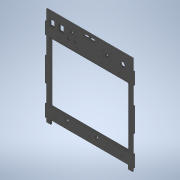
# Autodesk Inventor part: Frente Carcasa
Saved by Autodesk Inventor 2020 (Build 240168000, 168)
## iProperties
Created: 2020-06-04
Part Number: Frente Carcasa
Material: MDF Medium Density Fiberboard
Document SubType Name: Modeling
Designer: Dante
Density: 0.8 g/cm^3
Appearance: Gris oscuro
Mass: 813.806 g
Surface Area: 2644.18 cm^2
Volume: 1017.26 cm^3
Author: Dante
Autodesk Inventor part; units mm, degrees
ref_plane "YZ Plane" through (0, 0, 0) normal (1, 0, 0) x (0, 1, 0)
ref_plane "XZ Plane" through (0, 0, 0) normal (0, 1, 0) x (-1, 0, 0)
ref_plane "XY Plane" through (0, 0, 0) normal (0, 0, 1) x (1, 0, 0)
sketch "Sketch1" plane through (0, 0, 0) normal (0, 0, 1) x (1, 0, 0)
  line L0 (67.9652, 2.3975) -> (457.9652, 2.3975)
  line L1 (479.9652, -17.6025) -> (457.9652, -17.6025)
  line L2 (457.9652, -17.6025) -> (457.9652, 2.3975)
  line L3 (45.9652, -17.6025) -> (67.9652, -17.6025)
  line L4 (67.9652, -17.6025) -> (67.9652, 2.3975)
  line L5 (479.9652, 59.8925) -> (479.9652, 59.8925)
  line L6 (456.9652, 57.3975) -> (68.9652, 57.3975)
  line L7 (36.9652, 522.3965) -> (36.9552, 522.3965)
  line L8 (463.9652, 64.3975) -> (463.9652, 356.3975)
  line L9 (61.9652, 64.3975) -> (61.9652, 356.3975)
  line L10 (68.9652, 363.3975) -> (456.9652, 363.3975)
  line L11 (479.9652, 150.3975) -> (485.4652, 150.3975)
  line L12 (479.9652, 270.3975) -> (485.4652, 270.3975)
  line L13 (485.4652, 270.3975) -> (485.4652, 150.3975)
  line L14 (40.4652, 270.3975) -> (40.4652, 150.3975)
  line L15 (40.4652, 150.3975) -> (45.9652, 150.3975)
  line L16 (40.4652, 270.3975) -> (45.9652, 270.3975)
  circle A0 centre (95.9652, 27.3975) radius 3
  circle A1 centre (429.9652, 27.3975) radius 3
  circle A2 centre (417.4652, 381.0395) radius 3
  circle A3 centre (108.4652, 381.0395) radius 3
  circle A4 centre (327.4652, 381.0395) radius 3
  circle A5 centre (198.4652, 381.0395) radius 3
  circle A6 centre (262.9652, 27.3975) radius 3
  circle A7 centre (471.4652, 135.3975) radius 2
  circle A8 centre (471.4652, 285.3975) radius 2
  line L17 (45.9652, 270.3975) -> (45.9652, 360.3975)
  line L18 (45.9652, 360.3975) -> (40.4652, 360.3975)
  line L19 (40.4652, 360.3975) -> (40.4652, 420.3975)
  line L20 (40.4652, 420.3975) -> (45.9652, 420.3975)
  line L21 (45.9652, 475.4975) -> (45.9652, 420.3975)
  line L22 (45.9652, 360.3975) -> (45.9652, 270.3975)
  line L23 (45.9652, 150.3975) -> (45.9652, 60.3975)
  line L24 (45.9652, 60.3975) -> (40.4652, 60.3975)
  line L25 (40.4652, 60.3975) -> (40.4652, 0.3975)
  line L26 (40.4652, 0.3975) -> (45.9652, 0.3975)
  line L27 (45.9652, 150.3975) -> (45.9652, 60.3975)
  line L28 (45.9652, 0.3975) -> (45.9652, -17.6025)
  line L29 (479.9652, 360.3975) -> (485.4652, 360.3975)
  line L30 (485.4652, 360.3975) -> (485.4652, 420.3975)
  line L31 (485.4652, 420.3975) -> (479.9652, 420.3975)
  line L32 (479.9652, 475.4975) -> (479.9652, 420.3975)
  line L33 (479.9652, 150.3975) -> (479.9652, 60.3975)
  line L34 (479.9652, 60.3975) -> (485.4652, 60.3975)
  line L35 (485.4652, 60.3975) -> (485.4652, 0.3975)
  line L36 (485.4652, 0.3975) -> (479.9652, 0.3975)
  line L37 (479.9652, -17.6025) -> (479.9652, 0.3975)
  line L38 (479.9652, 60.3975) -> (479.9652, 150.3975)
  line L39 (479.9652, 270.3975) -> (479.9652, 360.3975)
  line L40 (262.9652, 474.8975) -> (262.9652, 460.6682)
  circle A9 centre (218.9652, 465.4975) radius 1.5
  circle A10 centre (218.9652, 400.4975) radius 1.5
  circle A11 centre (306.9652, 465.4975) radius 1.5
  circle A12 centre (306.9652, 400.4975) radius 1.5
  line L41 (266.4652, 463.3975) -> (290.7652, 463.3975)
  line L42 (290.7652, 463.3975) -> (290.7652, 450.7975)
  line L43 (290.7652, 450.7975) -> (266.4652, 450.7975)
  line L44 (266.4652, 450.7975) -> (266.4652, 463.3975)
  line L45 (235.4652, 463.3975) -> (259.7652, 463.3975)
  line L46 (259.7652, 463.3975) -> (259.7652, 450.7975)
  line L47 (259.7652, 450.7975) -> (235.4652, 450.7975)
  line L48 (235.4652, 450.7975) -> (235.4652, 463.3975)
  line L49 (86.9652, 440.4975) -> (65.4652, 440.4975)
  line L50 (65.4652, 440.4975) -> (65.4652, 414.9975)
  line L51 (65.4652, 414.9975) -> (86.9652, 414.9975)
  line L52 (86.9652, 414.9975) -> (86.9652, 440.4975)
  line L53 (87.0652, 441.9975) -> (87.0652, 413.4975)
  line L54 (65.3652, 413.4975) -> (65.3652, 441.9975)
  line L55 (133.4652, 440.4975) -> (111.9652, 440.4975)
  line L56 (111.9652, 440.4975) -> (111.9652, 414.9975)
  line L57 (111.9652, 414.9975) -> (133.4652, 414.9975)
  line L58 (133.4652, 414.9975) -> (133.4652, 440.4975)
  line L59 (133.5652, 441.9975) -> (133.5652, 413.4975)
  line L60 (111.8652, 413.4975) -> (111.8652, 441.9975)
  circle A13 centre (160.4652, 403.4975) radius 6
  circle A14 centre (175.4652, 435.4975) radius 6.5
  circle A15 centre (350.4652, 425.4975) radius 6.5
  circle A16 centre (193.4652, 448.4975) radius 2
  circle A17 centre (193.4652, 422.4975) radius 2
  circle A18 centre (157.4652, 448.4975) radius 2
  circle A19 centre (157.4652, 422.4975) radius 2
  circle A20 centre (368.4652, 438.4975) radius 2
  circle A21 centre (368.4652, 412.4975) radius 2
  circle A22 centre (332.4652, 438.4975) radius 2
  circle A23 centre (332.4652, 412.4975) radius 2
  circle A24 centre (429.9652, 425.4975) radius 11
  circle A25 centre (190.4652, 403.4975) radius 4.125
  line L61 (45.9652, 475.4975) -> (479.9652, 475.4975)
  line L62 (65.3652, 441.9975) -> (87.0652, 441.9975)
  line L63 (65.3652, 413.4975) -> (87.0652, 413.4975)
  line L64 (111.8652, 441.9975) -> (133.5652, 441.9975)
  line L65 (111.8652, 413.4975) -> (133.5652, 413.4975)
  arc A26 (68.9652, 363.3975) -> (61.9652, 356.3975) centre (68.9652, 356.3975) ccw
  arc A27 (61.9652, 64.3975) -> (68.9652, 57.3975) centre (68.9652, 64.3975) ccw
  arc A28 (456.9652, 57.3975) -> (463.9652, 64.3975) centre (456.9652, 64.3975) ccw
  arc A29 (463.9652, 356.3975) -> (456.9652, 363.3975) centre (456.9652, 356.3975) ccw
  line L66 (449.9652, 356.3975) -> (75.9652, 356.3975)
  line L67 (68.9652, 349.3975) -> (68.9652, 71.3975)
  line L68 (75.9652, 64.3975) -> (449.9652, 64.3975)
  line L69 (456.9652, 71.3975) -> (456.9652, 349.3975)
  arc A30 (75.9652, 356.3975) -> (68.9652, 349.3975) centre (75.9652, 349.3975) ccw
  arc A31 (456.9652, 349.3975) -> (449.9652, 356.3975) centre (449.9652, 349.3975) ccw
  arc A32 (449.9652, 64.3975) -> (456.9652, 71.3975) centre (449.9652, 71.3975) ccw
  arc A33 (68.9652, 71.3975) -> (75.9652, 64.3975) centre (75.9652, 71.3975) ccw
  circle A34 centre (471.4652, 217.4975) radius 2
  point P0 (77.9853, 6.3978)
  point P1 (463.9652, 475.4975)
  dimension "d148" = 55
  dimension "d187" = 434
  dimension "d211" = 168
  dimension "d212" = 5.5
  dimension "d214" = 5.5
  dimension "d218" = 120
  dimension "d220" = 6
  dimension "d229" = 6
  dimension "d234" = 6
  dimension "d235" = 6
  dimension "d238" = 6
  dimension "d239" = 6
  dimension "d243" = 4
  dimension "d245" = 4
  dimension "d247" = 150
  dimension "d248" = 153
  dimension "d254" = 90
  dimension "d256" = 90
  dimension "d257" = 90
  dimension "d258" = 60
  dimension "d259" = 90
  dimension "d260" = 5.5
  dimension "d261" = 60
  dimension "d262" = 90
  dimension "d263" = 5.5
  dimension "d264" = 60
  dimension "d265" = 90
  dimension "d266" = 60
  dimension "d267" = 120
  dimension "d270" = 3
  dimension "d271" = 44
  dimension "d273" = 3
  dimension "d274" = 65
  dimension "d275" = 88
  dimension "d283" = 24.3
  dimension "d284" = 3.5
  dimension "d285" = 24.3
  dimension "d286" = 3.2
  dimension "d288" = 12.6
  dimension "d289" = 12.6
  dimension "d290" = 68
  dimension "d291" = 68
  dimension "d298" = 25
  dimension "d299" = 21.5
  dimension "d300" = 25.5
  dimension "d302" = 21.5
  dimension "d303" = 25.5
  dimension "d305" = 25
  dimension "d307" = 12
  dimension "d311" = 13
  dimension "d333" = 22
  dimension "d334" = 22
  dimension "d437" = 13
  dimension "d440" = 4
  dimension "d441" = 13
  dimension "d442" = 4
  dimension "d444" = 18
  dimension "d445" = 4
  dimension "d446" = 18
  dimension "d447" = 4
  dimension "d448" = 13
  dimension "d449" = 18
  dimension "d450" = 4
  dimension "d451" = 4
  constraints: 140 end point, 35 centre point, 26 perpendicular, 19 parallel, 16 point on circle, 16 tangent, 11 horizontal, 7 vertical, 4 equal radius, 2 symmetric about line, 1 point on line, 5 other
  measures "d148" distance between parallel lines of L0 L6
  measures "d187" distance of L1.start L3.start
  measures "d211" distance of L1.start L11.start
  measures "d212" distance of L11.start L11.end
  measures "d214" distance of L12.start L12.end
  measures "d218" distance of L14.start L14.end
  measures "d220" diameter of A0
  measures "d229" diameter of A1
  measures "d234" diameter of A2
  measures "d235" diameter of A3
  measures "d238" diameter of A4
  measures "d239" diameter of A5
  measures "d243" diameter of A7
  measures "d245" diameter of A8
  measures "d247" distance of A7.centre A8.centre
  measures "d248" distance from line of L1 A7.centre
  measures "d254" distance of A2.centre A4.centre
  measures "d256" distance of A5.centre A3.centre
  measures "d257" distance of L16.end L17.end
  measures "d258" distance of L18.end L19.end
  measures "d259" distance of L15.end L23.end
  measures "d260" distance of L23.end L24.end
  measures "d261" distance of L24.end L25.end
  measures "d262" distance of L12.start L29.start
  measures "d263" distance of L29.start L29.end
  measures "d264" distance of L29.end L30.end
  measures "d265" distance of L11.start L33.end
  measures "d266" distance of L34.end L35.end
  measures "d267" distance of L12.end L11.end
  measures "d270" diameter of A9
  measures "d271" distance from line of A9.centre L40
  measures "d273" diameter of A10
  measures "d274" distance of A10.centre A9.centre
  measures "d275" distance of A10.centre A12.centre
  measures "d283" distance between parallel lines of L42 L44
  measures "d284" distance between parallel lines of L40 L44
  measures "d285" distance between parallel lines of L46 L48
  measures "d286" distance between parallel lines of L46 L40
  measures "d288" distance of L43.end L41.start
  measures "d289" distance of L45.end L47.start
  measures "d290" distance from line of L30 A2.centre
  measures "d291" distance from line of L19 A3.centre
  measures "d298" distance between parallel lines of L50 L19
  measures "d299" distance of L49.start L49.end
  measures "d300" distance of L51.end L49.start
  measures "d302" distance of L55.start L56.start
  measures "d303" distance of L57.end L55.start
  measures "d305" distance between parallel lines of L56 L52
  measures "d307" diameter of A13
  measures "d311" diameter of A14
  measures "d333" distance of L1.start L1.end
  measures "d334" distance of L3.start L4.start
  measures "d437" diameter of A15
  measures "d440" diameter of A16
  measures "d441" vertical distance of A16.centre A14.centre
  measures "d442" diameter of A17
  measures "d444" horizontal distance of A14.centre A16.centre
  measures "d445" diameter of A18
  measures "d446" horizontal distance of A18.centre A14.centre
  measures "d447" diameter of A19
  measures "d448" vertical distance of A19.centre A14.centre
  measures "d449" horizontal distance of A19.centre A14.centre
  measures "d450" diameter of A20
  measures "d451" diameter of A21
extrude "Extrusion6" add sketch "Sketch1" along normal blind 5.5 contours L4 L3 L28 L26 L25 L24 L23 L15 L14 L16 L17 L18 L19 L20 L21 L61 L32 L31 L30 L29 L39 L12 L13 L11 L33 L34 L35 L36 L37 L1 L2 L0
extrude "Extrusión9" add sketch "Sketch1" along normal blind 2.5 contours L6 A27 L9 A26 L10 A29 L8 A28
sketch "Boceto2" plane through (0, 0, 5.5) normal (0, 0, 1) x (1, 0, 0)
  line L0 (67.9652, 2.3975) -> (457.9652, 2.3975) projected
  circle A0 centre (150.9652, 40.3975) radius 7
  circle A1 centre (300.9652, 40.3975) radius 7
  line L1 (45.9652, 150.3975) -> (45.9652, 60.3975) projected
  line L2 (45.9652, 60.3975) -> (45.9652, 2.3975)
  dimension "d159" = 14
  dimension "d162" = 14
  dimension "d165" = 150
  dimension "d269" = 105
  constraints: 2 centre point, 2 end point, 1 vertical
  measures "d159" diameter of A0
  measures "d162" diameter of A1
  measures "d165" distance of A1.centre A0.centre
  measures "d269" distance from line of L2 A0.centre
extrude "Extrusión10" cut sketch "Boceto2" against normal blind 9
body "Solid3"
